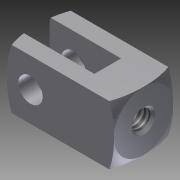
# Autodesk Inventor part: D-26646
Saved by Autodesk Inventor 2012 (Build 160160000, 160)
## iProperties
Created: 2013-01-17
Part Number: D-26646
Material: Default
Catalog Web Link: www.cadenas.de
Description: Piston Rod Clevis for Original Line Cylinders - Body-
Vendor: BIMBA
Document SubType Name: Modeling
Designer: William
Manufacturer: BIMBA
Density: 1 g/cm^3
Category: PARTsolutions
Company: BIMBA
Title: D-26646
Author: Cadenas PARTsolutions
PSOL_IDENT_0: {\\10.0.0.242\data_v9\23d-libs\bimba\bimba\bimba_imperial\bimba_full_line\original_line_cylinders\ac
PSOL_IDENT_1: cessories\piston_rod_clevis_body.prj},202 {VTYP=3D},{NB=D-26646},{LINA=D-26646},{NN=Piston Rod Clevi
PSOL_IDENT_2: s for Original Line Cylinders - Body},{DATE=06.12.2012 09:37:17},{GEOMDATE=06.12.2012 07:16:06},{VER
PSOL_IDENT_3: SION=},{LINEID=10},{LINESUBID=-1},{WBVAR=}  {NB=D-26646},{LINA=D-26646},{KT=DUMMY},{PN=D-26646},{L=0
PSOL_IDENT_4: .56200000},{L1=0.43800000},{L2=0.18800000},{W=0.14000000},{W1=0.31000000},{DIA1=0.12750000},{DIA1CS=
PSOL_IDENT_5: 0.00000000},{DIA2=0.31200000},{DIA3=0.09950000},{CS=90.00000000},{CDP=0.02000000},{AN=30.00000000},{
PSOL_IDENT_6: NDM=0.12500000},{CODE=UNC},{NDMDP=0.18000000},{COLOR=0.75,0.75,0.75,0.00}
CNS_NB: D-26646
CNS_NBSYN: $PN.
CNS_LINA: D-26646
CNS_PN: D-26646
CNS_L: 0.56200000
CNS_L1: 0.43800000
CNS_L2: 0.18800000
CNS_W: 0.14000000
CNS_W1: 0.31000000
CNS_DIA1: 0.12750000
CNS_DIA1CS: 0.00000000
CNS_DIA2: 0.31200000
CNS_DIA3: 0.09950000
CNS_CS: 90.00000000
CNS_CDP: 0.02000000
CNS_AN: 30.00000000
CNS_NDM: 0.12500000
CNS_CODE: UNC
CNS_NDMDP: 0.18000000
CNS_COLOR: 0.75,0.75,0.75,0.00
SUPPLIER: BIMBA
ARTICLENO: D-26646
BOMINFO: D-26646
CREATOR: CADENAS GmbH
Autodesk Inventor part; units mm, degrees
sketch "Sketch_1" plane through (0, 0, 0) normal (0, 0, 1) x (1, 0, 0)
  line L0 (-3.1496, 3.937) -> (-3.1496, -3.937)
  line L1 (-3.1496, -3.937) -> (11.1252, -3.937)
  line L2 (11.1252, -3.937) -> (11.1252, 3.937)
  line L3 (11.1252, 3.937) -> (-3.1496, 3.937)
  constraints: 8 end point
extrude "Extrusion1" add sketch "Sketch_1" along normal mid plane 7.874
sketch "Sketch_2" plane through (0, 0, 0) normal (0, 1, 0) x (-1, 0, 0)
  line L0 (3.1496, -1.778) -> (3.1496, 1.778)
  line L1 (3.1496, 1.778) -> (-6.35, 1.778)
  line L2 (-6.35, 1.778) -> (-6.35, -1.778)
  line L3 (-6.35, -1.778) -> (3.1496, -1.778)
  constraints: 8 end point
extrude "Extrusion2" cut sketch "Sketch_2" along normal mid plane 7.874
sketch "Sketch3" plane through (11.1252, -3.937, 3.937) normal (1, 0, 0) x (0, 0, -1)
  point P0 (3.937, 3.937)
hole "Drilling 1" at (11.1252, 0, 0) direction (-1, 0, 0) diameter 2.4867 depth 4.572 countersink diameter 3.175 countersink angle 90 thread size "5-40 UNC" class "2B" standard "ANSI Unified Screw Threads"
sketch "Sketch4" plane through (6.5532, 0, 0) normal (1, 0, 0) x (0, 0, -1)
  point P0 (0, 0)
hole "Drilling 2" at (6.5532, 0, 0) direction (-1, 0, 0) diameter 2.5273 depth 0.2032
sketch "Sketch5" plane through (0, 0, -3.937) normal (0, 0, -1) x (-1, 0, 0)
  point P0 (0, 0)
hole "Drilling 3" at (0, 0, -3.937) direction (0, 0, 1) diameter 3.2385 depth 7.874
sketch "Sketch_9" plane through (0, 0, 0) normal (0, 0, 1) x (1, 0, 0)
  line L0 (15.0622, 0) -> (11.1252, 0)
  line L1 (11.1252, 0) -> (11.1252, 3.937)
  arc A0 (11.1252, 3.937) -> (8.5852, 7.874) centre (3.7528, 1.9685) ccw
  line L2 (8.5852, 7.874) -> (15.0622, 7.874)
  line L3 (15.0622, 7.874) -> (15.0622, 0)
  line L4 (15.0622, 0) -> (11.1252, 0)
  constraints: 10 end point, 2 point on circle, 1 centre point
revolve "Revolution1" cut sketch "Sketch_9" angle 360 about axis through (15.0622, 0, 0) along (1, 0, 0)
sketch "Sketch_10" plane through (0, 0, 0) normal (0, 0, 1) x (1, 0, 0)
  line L0 (-3.1496, 0) -> (-7.0866, 0)
  line L1 (-7.0866, 0) -> (-7.0866, 7.874)
  line L2 (-7.0866, 7.874) -> (-0.6096, 7.874)
  arc A0 (-0.6096, 7.874) -> (-3.1496, 3.937) centre (4.2228, 1.9685) ccw
  line L3 (-3.1496, 3.937) -> (-3.1496, 0)
  line L4 (-3.1496, 0) -> (-7.0866, 0)
  constraints: 10 end point, 2 point on circle, 1 centre point
revolve "Revolution2" cut sketch "Sketch_10" angle 360 about axis through (-3.1496, 0, 0) along (1, 0, 0)
ref_plane "th1_XY" through (11.1252, 1.5875, 0) normal (0, 0, 1) x (1, 0, 0)
ref_plane "th1_YZ" through (11.1252, 1.5875, 0) normal (1, 0, 0) x (0, 1, 0)
ref_plane "th1_ZX" through (11.1252, 1.5875, 0) normal (0, 1, 0) x (0, 0, 1)
ref_plane "th2_XY" through (11.1252, -1.5875, 0) normal (0, 0, 1) x (1, 0, 0)
ref_plane "th2_YZ" through (11.1252, -1.5875, 0) normal (1, 0, 0) x (0, 1, 0)
ref_plane "th2_ZX" through (11.1252, -1.5875, 0) normal (0, 1, 0) x (0, 0, 1)
ref_plane "rod_clevis_body_XY" through (0, 0, 0) normal (0, 0, 1) x (1, 0, 0)
ref_plane "rod_clevis_body_YZ" through (0, 0, 0) normal (1, 0, 0) x (0, 1, 0)
ref_plane "rod_clevis_body_ZX" through (0, 0, 0) normal (0, 1, 0) x (0, 0, 1)
ref_plane "piston_rod_clevis_XY" through (11.1252, 0, 0) normal (1, 0, 0) x (0, 0, -1)
ref_plane "piston_rod_clevis_YZ" through (11.1252, 0, 0) normal (0, 0, -1) x (0, 1, 0)
ref_plane "piston_rod_clevis_ZX" through (11.1252, 0, 0) normal (0, 1, 0) x (1, 0, 0)
ref_plane "dummy_XY" through (0, 0, 0) normal (0, 0, 1) x (1, 0, 0)
ref_plane "dummy_YZ" through (0, 0, 0) normal (1, 0, 0) x (0, 1, 0)
ref_plane "dummy_ZX" through (0, 0, 0) normal (0, 1, 0) x (0, 0, 1)
ref_plane "l11_XY" through (11.1252, 3.937, 0) normal (0, 0, 1) x (1, 0, 0)
ref_plane "l11_YZ" through (11.1252, 3.937, 0) normal (1, 0, 0) x (0, 1, 0)
ref_plane "l11_ZX" through (11.1252, 3.937, 0) normal (0, 1, 0) x (0, 0, 1)
ref_plane "l12_XY" through (0, 3.937, 0) normal (0, 0, 1) x (1, 0, 0)
ref_plane "l12_YZ" through (0, 3.937, 0) normal (1, 0, 0) x (0, 1, 0)
ref_plane "l12_ZX" through (0, 3.937, 0) normal (0, 1, 0) x (0, 0, 1)
ref_plane "l1_XY" through (11.1252, 3.937, 0) normal (0, 0, 1) x (1, 0, 0)
ref_plane "l1_YZ" through (11.1252, 3.937, 0) normal (1, 0, 0) x (0, 1, 0)
ref_plane "l1_ZX" through (11.1252, 3.937, 0) normal (0, 1, 0) x (0, 0, 1)
ref_plane "h1_XY" through (-3.1496, 3.937, 0) normal (0, 0, 1) x (1, 0, 0)
ref_plane "h1_YZ" through (-3.1496, 3.937, 0) normal (1, 0, 0) x (0, 1, 0)
ref_plane "h1_ZX" through (-3.1496, 3.937, 0) normal (0, 1, 0) x (0, 0, 1)
ref_plane "l2_XY" through (-3.1496, 3.937, 0) normal (0, 0, 1) x (1, 0, 0)
ref_plane "l2_YZ" through (-3.1496, 3.937, 0) normal (1, 0, 0) x (0, 1, 0)
ref_plane "l2_ZX" through (-3.1496, 3.937, 0) normal (0, 1, 0) x (0, 0, 1)
ref_plane "h2_XY" through (-3.1496, -3.937, 0) normal (0, 0, 1) x (1, 0, 0)
ref_plane "h2_YZ" through (-3.1496, -3.937, 0) normal (1, 0, 0) x (0, 1, 0)
ref_plane "h2_ZX" through (-3.1496, -3.937, 0) normal (0, 1, 0) x (0, 0, 1)
ref_plane "w11_XY" through (-3.1496, 0, -1.778) normal (0, 1, 0) x (1, 0, 0)
ref_plane "w11_YZ" through (-3.1496, 0, -1.778) normal (1, 0, 0) x (0, 0, -1)
ref_plane "w11_ZX" through (-3.1496, 0, -1.778) normal (0, 0, -1) x (0, 1, 0)
ref_plane "w12_XY" through (-3.1496, 0, 1.778) normal (0, 1, 0) x (1, 0, 0)
ref_plane "w12_YZ" through (-3.1496, 0, 1.778) normal (1, 0, 0) x (0, 0, -1)
ref_plane "w12_ZX" through (-3.1496, 0, 1.778) normal (0, 0, -1) x (0, 1, 0)
ref_plane "l21_XY" through (11.1252, 0, 0) normal (0, 1, 0) x (1, 0, 0)
ref_plane "l21_YZ" through (11.1252, 0, 0) normal (1, 0, 0) x (0, 0, -1)
ref_plane "l21_ZX" through (11.1252, 0, 0) normal (0, 0, -1) x (0, 1, 0)
ref_plane "l22_XY" through (6.35, 0, 0) normal (0, 1, 0) x (1, 0, 0)
ref_plane "l22_YZ" through (6.35, 0, 0) normal (1, 0, 0) x (0, 0, -1)
ref_plane "l22_ZX" through (6.35, 0, 0) normal (0, 0, -1) x (0, 1, 0)
ref_plane "w1_XY" through (11.1252, 0, -3.937) normal (0, 1, 0) x (1, 0, 0)
ref_plane "w1_YZ" through (11.1252, 0, -3.937) normal (1, 0, 0) x (0, 0, -1)
ref_plane "w1_ZX" through (11.1252, 0, -3.937) normal (0, 0, -1) x (0, 1, 0)
ref_plane "w2_XY" through (11.1252, 0, 3.937) normal (0, 1, 0) x (1, 0, 0)
ref_plane "w2_YZ" through (11.1252, 0, 3.937) normal (1, 0, 0) x (0, 0, -1)
ref_plane "w2_ZX" through (11.1252, 0, 3.937) normal (0, 0, -1) x (0, 1, 0)
ref_plane "to_cylinder_XY" through (6.35, 0, 0) normal (1, 0, 0) x (0, 0, -1)
ref_plane "to_cylinder_YZ" through (6.35, 0, 0) normal (0, 0, -1) x (0, 1, 0)
ref_plane "to_cylinder_ZX" through (6.35, 0, 0) normal (0, 1, 0) x (1, 0, 0)
body "Solid1"
